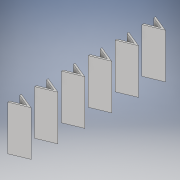
# Autodesk Inventor part: 45deg_20mm
Saved by Autodesk Inventor 2019 (Build 230136000, 136)
## iProperties
Created: 2019-03-12
Part Number: 45deg_20mm
Material: Generic
Document SubType Name: Modeling
Designer: erwin
Density: 1 g/cm^3
Appearance: Default
Author: erwin
Autodesk Inventor part; units mm, degrees
ref_plane "YZ Plane" through (0, 0, 0) normal (1, 0, 0) x (0, 1, 0)
ref_plane "XZ Plane" through (0, 0, 0) normal (0, 1, 0) x (-1, 0, 0)
ref_plane "XY Plane" through (0, 0, 0) normal (0, 0, 1) x (1, 0, 0)
sketch "Sketch1" plane through (0, 0, 0) normal (0, 1, 0) x (-1, 0, 0)
  line L0 (0, 0) -> (-18.4776, -7.6537)
  line L1 (-18.4776, -7.6537) -> (0, -15.3073)
  line L2 (0, -15.3073) -> (0, -13.3073)
  line L3 (0, -13.3073) -> (-13.6492, -7.6537)
  line L4 (-13.6492, -7.6537) -> (0, -2)
  line L5 (0, -2) -> (0, 0)
  dimension "d0" = 2
  dimension "d1" = 20
  dimension "d2" = 45
  constraints: 12 end point, 2 equal length, 2 parallel, 1 collinear, 1 point on line, 1 vertical
  measures "d0" distance of L4.end L0.start
  measures "d1" distance of L0.start L0.end
  measures "d2" angle of L3 L4
extrude "Extrusion1" add sketch "Sketch1" along normal blind 50
pattern_linear "Rectangular Pattern1" count 6 spacing 30 along (0, 0, 1) of "Extrusion1"
body "Solid1"
